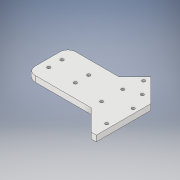
# Autodesk Inventor part: MotorSuspension
Saved by Autodesk Inventor 2018 (Build 220112000, 112)
## iProperties
Created: 2018-08-27
Part Number: MotorSuspension
Material: Generic
Document SubType Name: Modeling
Designer: anirudh
Density: 1 g/cm^3
Appearance: White
Author: anirudh
Autodesk Inventor part; units mm, degrees
ref_plane "YZ Plane" through (0, 0, 0) normal (1, 0, 0) x (0, 1, 0)
ref_plane "XZ Plane" through (0, 0, 0) normal (0, 1, 0) x (-1, 0, 0)
ref_plane "XY Plane" through (0, 0, 0) normal (0, 0, 1) x (1, 0, 0)
sketch "Sketch1" plane through (0, 0, 0) normal (0, 1, 0) x (-1, 0, 0)
  line L0 (0, 0) -> (67.2338, 0)
  arc A0 (76.7588, -9.525) -> (67.2338, 0) centre (67.2338, -9.525) ccw
  arc A1 (67.2338, -48.9204) -> (76.7588, -39.3954) centre (67.2338, -39.3954) ccw
  line L1 (76.7588, -9.525) -> (76.7588, -39.3954)
  line L2 (67.2338, -48.9204) -> (15.367, -48.9204)
  line L3 (15.367, -48.9204) -> (-3.6891, -67.9765)
  line L4 (0, 0) -> (-25.3962, 25.3962)
  circle A2 centre (35.2298, -16.4592) radius 1.905
  circle A3 centre (35.2298, -32.4612) radius 1.905
  circle A4 centre (67.2338, -32.4612) radius 1.905
  circle A5 centre (67.2338, -16.4592) radius 1.905
  circle A6 centre (-26.1112, -24.4602) radius 1.85
  circle A7 centre (-26.1112, 7.2898) radius 1.85
  line L5 (-25.3962, 25.3962) -> (-31.7462, 25.3962)
  line L6 (-31.7462, 25.3962) -> (-31.7462, -39.9194)
  line L7 (-31.7462, -39.9194) -> (-3.6891, -67.9765)
  circle A8 centre (0, -12.7) radius 1.85
  circle A9 centre (0, -38.1) radius 1.85
  line L8 (-3.6891, -67.9765) -> (-12.6694, -58.9962)
  circle A10 centre (-3.6891, -59.4929) radius 1.85
  circle A11 centre (-17.1882, -44.4383) radius 1.85
  dimension "d21" = 6.35
  constraints: 18 end point, 12 centre point, 4 point on circle, 3 horizontal, 2 perpendicular, 1 point on line, 1 vertical
  measures "d21" distance of L4.end L5.end
extrude "Extrusion1" add sketch "Sketch1" along normal blind 7
body "Solid1"
